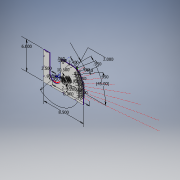
# Autodesk Inventor part: BB Gun Angle Adjustmeter
Saved by Autodesk Inventor 2018 (Build 220112000, 112)
## iProperties
Created: 2019-05-22
Part Number: BB Gun Angle Adjustmeter
Material: Generic
Document SubType Name: Modeling
Designer: 871357
Density: 1 g/cm^3
Appearance: Default
Author: 871357
Autodesk Inventor part; units mm, degrees
ref_plane "YZ Plane" through (0, 0, 0) normal (1, 0, 0) x (0, 1, 0)
ref_plane "XZ Plane" through (0, 0, 0) normal (0, 1, 0) x (-1, 0, 0)
ref_plane "XY Plane" through (0, 0, 0) normal (0, 0, 1) x (1, 0, 0)
sketch "Sketch1" plane through (0, 0, 0) normal (0, 0, 1) x (1, 0, 0)
  line L0 (0, 0) -> (215.9, 0)
  line L1 (0, 152.4) -> (0, 0)
  line L2 (33.02, 152.4) -> (33.02, 55.88)
  arc A0 (33.02, 55.88) -> (93.98, 55.88) centre (63.5, 55.88) ccw
  line L3 (93.98, 55.88) -> (93.98, 152.4)
  line L4 (63.5, 55.88) -> (215.9, 55.88) construction
  line L5 (63.5, 55.88) -> (202.5207, 68.0427) construction
  line L6 (63.5, 55.88) -> (203.0517, 55.88) construction
  line L7 (63.5, 55.88) -> (200.4952, 80.036) construction
  line L8 (63.5, 55.88) -> (202.6086, 55.88) construction
  line L9 (63.5, 55.88) -> (197.1611, 91.6944) construction
  line L10 (63.5, 55.88) -> (201.8761, 55.88) construction
  line L11 (63.5, 55.88) -> (192.5792, 102.861) construction
  line L12 (63.5, 55.88) -> (200.8632, 55.88) construction
  line L13 (63.5, 55.88) -> (167.1672, 159.5472) construction
  line L14 (63.5, 55.88) -> (210.1076, 55.88) construction
  line L15 (63.5, 55.88) -> (201.6213, 120.287) construction
  line L16 (63.5, 55.88) -> (215.9, 55.88) construction
  line L17 (63.5, 55.88) -> (185.723, 141.4615) construction
  line L18 (63.5, 55.88) -> (212.7067, 55.88) construction
  line L19 (63.5, 55.88) -> (195.0554, 131.8335) construction
  line L20 (63.5, 55.88) -> (215.4071, 55.88) construction
  line L21 (63.5, 55.88) -> (173.8375, 148.4642) construction
  line L22 (63.5, 55.88) -> (207.5354, 55.88) construction
  line L23 (39.37, 55.88) -> (87.63, 55.88) construction
  arc A1 (39.37, 55.88) -> (87.63, 55.88) centre (63.5, 55.88) ccw construction
  arc A2 (184.577, 0) -> (155.5115, 152.4) centre (63.5, 55.88) ccw construction
  line L24 (67.3948, 25.6499) -> (219.7948, 178.0499) construction
  line L25 (51.758, 27.7525) -> (525.7284, 154.7525) construction
  line L26 (54.2541, 26.8362) -> (472.9697, 179.2362) construction
  line L27 (47.0521, 30.2188) -> (627.6987, 81.0188) construction
  line L28 (64.7453, 25.4254) -> (246.3685, 177.8254) construction
  line L29 (49.3512, 28.8829) -> (625.5534, 130.4829) construction
  line L30 (56.8206, 26.1409) -> (383.6435, 178.5409) construction
  line L31 (62.0863, 25.4328) -> (279.736, 177.8328) construction
  line L32 (59.438, 25.6719) -> (323.4025, 178.0719) construction
  line L33 (44.8781, 31.75) -> (248.0781, 31.75) construction
  line L34 (179.4762, 121.6961) -> (182.9052, 121.6961)
  line L35 (182.9052, 121.6961) -> (182.9052, 118.2671)
  line L36 (182.9052, 118.2671) -> (179.4762, 118.2671)
  line L37 (179.4762, 118.2671) -> (179.4762, 121.6961)
  line L38 (184.7711, 111.3376) -> (188.2001, 111.3376)
  line L39 (188.2001, 111.3376) -> (188.2001, 107.9086)
  line L40 (188.2001, 107.9086) -> (184.7711, 107.9086)
  line L41 (184.7711, 107.9086) -> (184.7711, 111.3376)
  line L42 (189.1431, 100.5571) -> (192.5721, 100.5571)
  line L43 (192.5721, 100.5571) -> (192.5721, 97.1281)
  line L44 (192.5721, 97.1281) -> (189.1431, 97.1281)
  line L45 (189.1431, 97.1281) -> (189.1431, 100.5571)
  line L46 (192.5588, 89.4366) -> (195.9878, 89.4366)
  line L47 (195.9878, 89.4366) -> (195.9878, 86.0076)
  line L48 (195.9878, 86.0076) -> (192.5588, 86.0076)
  line L49 (192.5588, 86.0076) -> (192.5588, 89.4366)
  line L50 (194.9924, 78.0607) -> (198.4214, 78.0607)
  line L51 (198.4214, 78.0607) -> (198.4214, 74.6317)
  line L52 (198.4214, 74.6317) -> (194.9924, 74.6317)
  line L53 (194.9924, 74.6317) -> (194.9924, 78.0607)
  line L54 (196.4252, 66.516) -> (199.8542, 66.516)
  line L55 (199.8542, 66.516) -> (199.8542, 63.087)
  line L56 (199.8542, 63.087) -> (196.4252, 63.087)
  line L57 (196.4252, 63.087) -> (196.4252, 66.516)
  line L58 (196.8463, 54.8903) -> (200.2753, 54.8903)
  line L59 (200.2753, 54.8903) -> (200.2753, 51.4613)
  line L60 (200.2753, 51.4613) -> (196.8463, 51.4613)
  line L61 (196.8463, 51.4613) -> (196.8463, 54.8903)
  line L62 (196.2526, 43.2722) -> (199.6816, 43.2722)
  line L63 (199.6816, 43.2722) -> (199.6816, 39.8432)
  line L64 (199.6816, 39.8432) -> (196.2526, 39.8432)
  line L65 (196.2526, 39.8432) -> (196.2526, 43.2722)
  line L66 (194.6486, 31.75) -> (198.0776, 31.75)
  line L67 (198.0776, 31.75) -> (198.0776, 28.321)
  line L68 (198.0776, 28.321) -> (194.6486, 28.321)
  line L69 (194.6486, 28.321) -> (194.6486, 31.75)
  line L70 (173.2986, 131.5536) -> (176.7276, 131.5536)
  line L71 (176.7276, 131.5536) -> (176.7276, 128.1246)
  line L72 (176.7276, 128.1246) -> (173.2986, 128.1246)
  line L73 (173.2986, 128.1246) -> (173.2986, 131.5536)
  arc A3 (215.9, 55.88) -> (199.5976, 124.46) centre (63.5, 55.88) ccw
  line L74 (215.9, 0) -> (215.9, 58.25)
  line L75 (215.9, 152.2593) -> (215.9, 152.4)
  arc A4 (199.5976, 124.46) -> (154.2317, 152.4) centre (154.2317, 101.6) ccw
  line L76 (154.2317, 152.4) -> (93.98, 152.4)
  line L77 (33.02, 152.4) -> (0, 152.4)
  line L78 (81.2098, 125.6753) -> (148.8905, 193.356) construction
  line L79 (95.25, 152.4) -> (102.87, 152.4)
  line L80 (102.87, 152.4) -> (102.87, 148.59)
  line L81 (102.87, 148.59) -> (95.25, 148.59)
  line L82 (95.25, 148.59) -> (95.25, 152.4)
  point P0 (181.4392, 152.4)
  dimension "d1" = 30.48
  dimension "d22" = 266.7
  dimension "d2" = 215.9
  dimension "d3" = 152.4
  dimension "d4" = 55.88
  dimension "d5" = 0
  dimension "d6" = 5
  dimension "d7" = 10
  dimension "d8" = 15
  dimension "d9" = 20
  dimension "d10" = 45
  dimension "d11" = 63.5
  dimension "d12" = 25
  dimension "d13" = 35
  dimension "d14" = 30
  dimension "d15" = 40
  dimension "d16" = 45
  dimension "d19" = 24.13
  dimension "d21" = 0
  dimension "d23" = 24.13
  dimension "d26" = 24.13
  dimension "d28" = 24.13
  dimension "d30" = 24.13
  dimension "d32" = 24.13
  dimension "d34" = 24.13
  dimension "d36" = 24.13
  dimension "d38" = 24.13
  dimension "d39" = 24.13
  dimension "d41" = 203.2
  dimension "d42" = 3.429
  dimension "d43" = 3.429
  dimension "d44" = 3.429
  dimension "d45" = 3.429
  dimension "d46" = 3.429
  dimension "d47" = 3.429
  dimension "d48" = 3.429
  dimension "d49" = 3.429
  dimension "d50" = 3.429
  dimension "d51" = 3.429
  dimension "d52" = 3.429
  dimension "d53" = 3.429
  dimension "d54" = 3.429
  dimension "d55" = 3.429
  dimension "d56" = 3.429
  dimension "d57" = 3.429
  dimension "d58" = 3.429
  dimension "d59" = 3.429
  dimension "d60" = 3.429
  dimension "d61" = 3.429
  dimension "d62" = 50.8
  dimension "d82" = 60.96
  dimension "d83" = 7.62
  dimension "d84" = 3.81
  dimension "d85" = 1.27
  constraints: 166 end point, 37 parallel, 21 horizontal, 16 point on line, 13 perpendicular, 11 point on circle, 9 equal length, 4 tangent, 4 vertical, 3 centre point, 2 coincident, 1 line through centre, 28 other
  measures "d2" distance of L0.start L0.end
  measures "d3" distance of L1.start L0.start
  measures "d4" distance from line of L0 L4.start
  measures "d5" vertical distance of L4.end L4.start
  measures "d6" angle of L6 L5
  measures "d7" angle of L8 L7
  measures "d8" angle of L10 L9
  measures "d9" angle of L12 L11
  measures "d10" angle of L14 L13
  measures "d11" distance from line of L1 L4.start
  measures "d12" angle of L16 L15
  measures "d13" angle of L18 L17
  measures "d14" angle of L20 L19
  measures "d15" angle of L22 L21
  measures "d16" angle of L20 L13
  measures "d19" radius of A1
  measures "d21" distance of L4.start A1.centre
  measures "d23" distance between parallel lines of L13 L24
  measures "d26" distance between parallel lines of L21 L28
  measures "d28" distance between parallel lines of L17 L31
  measures "d30" distance between parallel lines of L19 L32
  measures "d32" distance between parallel lines of L15 L30
  measures "d34" distance between parallel lines of L11 L26
  measures "d36" distance between parallel lines of L9 L25
  measures "d38" distance between parallel lines of L7 L29
  measures "d39" distance between parallel lines of L5 L27
  measures "d41" distance of L33.start L33.end
  measures "d42" distance of L35.end L36.end
  measures "d43" distance of L34.end L35.end
  measures "d44" distance of L39.end L40.end
  measures "d45" distance of L38.end L39.end
  measures "d46" distance of L43.end L44.end
  measures "d47" distance of L42.end L43.end
  measures "d48" distance of L47.end L48.end
  measures "d49" distance of L46.end L47.end
  measures "d50" distance of L51.end L52.end
  measures "d51" distance of L50.end L51.end
  measures "d52" distance of L55.end L56.end
  measures "d53" distance of L54.end L55.end
  measures "d54" distance of L59.end L60.end
  measures "d55" distance of L58.end L59.end
  measures "d56" distance of L63.end L64.end
  measures "d57" distance of L62.end L63.end
  measures "d58" distance of L67.end L68.end
  measures "d59" distance of L66.end L67.end
  measures "d60" distance of L71.end L72.end
  measures "d61" distance of L70.end L71.end
  measures "d62" radius of A4
  measures "d82" distance between parallel lines of L24 L78
  measures "d83" distance of L80.end L81.end
  measures "d84" distance of L79.end L80.end
  measures "d85" distance between parallel lines of L82 L3
extrude "Extrusion1" add sketch "Sketch1" along normal blind 2.54
sketch "Sketch2" plane through (0, 0, 2.54) normal (0, 0, 1) x (1, 0, 0)
  line L0 (0, 152.4) -> (0, 0) projected
  line L1 (0, 25.4) -> (3.81, 25.4)
  line L2 (3.81, 25.4) -> (3.81, 33.02)
  line L3 (3.81, 33.02) -> (0, 33.02)
  line L4 (0, 33.02) -> (0, 25.4)
  line L5 (0, 0) -> (215.9, 0) projected
  line L6 (0, 127) -> (3.81, 127)
  line L7 (3.81, 127) -> (3.81, 119.38)
  line L8 (3.81, 119.38) -> (0, 119.38)
  line L9 (0, 119.38) -> (0, 127)
  line L10 (33.02, 152.4) -> (0, 152.4) projected
  line L11 (0, 71.12) -> (3.81, 71.12)
  line L12 (3.81, 71.12) -> (3.81, 78.74)
  line L13 (3.81, 78.74) -> (0, 78.74)
  line L14 (0, 78.74) -> (0, 71.12)
  line L15 (38.1, 0) -> (45.72, 0)
  line L16 (45.72, 0) -> (45.72, 3.81)
  line L17 (45.72, 3.81) -> (38.1, 3.81)
  line L18 (38.1, 3.81) -> (38.1, 0)
  line L19 (177.8, 0) -> (170.18, 0)
  line L20 (170.18, 0) -> (170.18, 3.81)
  line L21 (170.18, 3.81) -> (177.8, 3.81)
  line L22 (177.8, 3.81) -> (177.8, 0)
  line L23 (215.9, 0) -> (215.9, 55.88) projected
  line L24 (104.14, 0) -> (111.76, 0)
  line L25 (111.76, 0) -> (111.76, 3.81)
  line L26 (111.76, 3.81) -> (104.14, 3.81)
  line L27 (104.14, 3.81) -> (104.14, 0)
  line L28 (102.87, 148.59) -> (95.25, 148.59) projected
  line L29 (95.25, 148.59) -> (95.25, 152.4) projected
  line L30 (154.2317, 152.4) -> (93.98, 152.4) projected
  line L31 (102.87, 152.4) -> (102.87, 148.59) projected
  line L32 (95.25, 152.4) -> (102.87, 152.4)
  line L33 (102.87, 152.4) -> (102.87, 148.59)
  line L34 (102.87, 148.59) -> (95.25, 148.59)
  line L35 (95.25, 148.59) -> (95.25, 152.4)
  line L36 (12.7, 152.4) -> (20.32, 152.4)
  line L37 (20.32, 152.4) -> (20.32, 148.59)
  line L38 (20.32, 148.59) -> (12.7, 148.59)
  line L39 (12.7, 148.59) -> (12.7, 152.4)
  dimension "d65" = 3.81
  dimension "d66" = 7.62
  dimension "d67" = 25.4
  dimension "d68" = 7.62
  dimension "d69" = 25.4
  dimension "d70" = 3.81
  dimension "d71" = 7.62
  dimension "d72" = 38.1
  dimension "d73" = 7.62
  dimension "d74" = 3.81
  dimension "d75" = 38.1
  dimension "d76" = 7.62
  dimension "d77" = 3.81
  dimension "d78" = 38.1
  dimension "d79" = 7.62
  dimension "d80" = 3.81
  dimension "d81" = 58.42
  dimension "d86" = 7.62
  dimension "d87" = 3.81
  dimension "d88" = 12.7
  dimension "d89" = 3.81
  constraints: 64 end point, 16 parallel, 8 horizontal, 8 perpendicular, 7 point on line
  measures "d65" distance of L1.start L1.end
  measures "d66" distance of L1.end L2.end
  measures "d67" distance between parallel lines of L5 L1
  measures "d68" distance of L6.end L7.end
  measures "d69" distance between parallel lines of L10 L6
  measures "d70" distance of L13.end L12.end
  measures "d71" distance of L12.end L11.end
  measures "d72" distance between parallel lines of L3 L11
  measures "d73" distance of L17.end L16.end
  measures "d74" distance of L16.end L15.end
  measures "d75" distance between parallel lines of L0 L18
  measures "d76" distance of L20.end L21.end
  measures "d77" distance of L19.end L20.end
  measures "d78" distance between parallel lines of L23 L22
  measures "d79" distance of L26.end L25.end
  measures "d80" distance of L25.end L24.end
  measures "d81" distance between parallel lines of L27 L16
  measures "d86" distance of L37.end L38.end
  measures "d87" distance of L36.end L37.end
  measures "d88" distance between parallel lines of L0 L39
  measures "d89" distance of L7.end L8.end
extrude "Extrusion2" cut sketch "Sketch2" against normal blind 25.4
body "Solid1"
